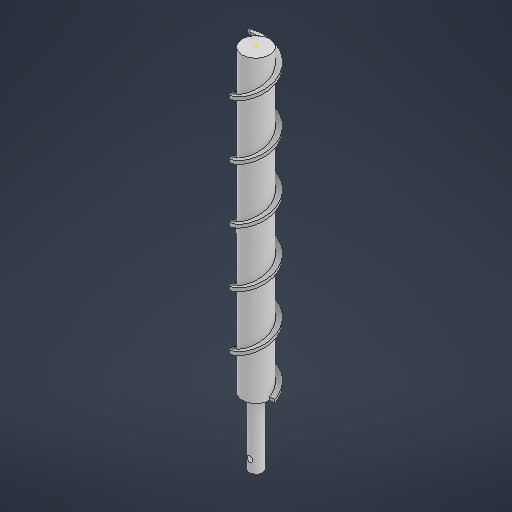
# Autodesk Inventor part: alimentaciion tornillo
Saved by Autodesk Inventor 2026.1 (Build 301233020, 233B)
## iProperties
Created: 2025-12-02
Part Number: alimentaciion tornillo
Material: Genérico
Document SubType Name: Modeling
Designer: benja
Density: 1 g/cm^3
Appearance: Valor por defecto
Author: benja
Autodesk Inventor part; units mm, degrees
ref_plane "YZ Plane" through (0, 0, 0) normal (1, 0, 0) x (0, 1, 0)
ref_plane "XZ Plane" through (0, 0, 0) normal (0, 1, 0) x (-1, 0, 0)
ref_plane "XY Plane" through (0, 0, 0) normal (0, 0, 1) x (1, 0, 0)
sketch "Boceto1" plane through (0, 0, 0) normal (0, 1, 0) x (-1, 0, 0)
  circle A0 centre (0, 0) radius 12.5
  dimension "d0" = 25
  constraints: 1 centre point, 1 coincident
  measures "d0" diameter of A0
extrude "Extrusión1" add sketch "Boceto1" along normal blind 271.2
sketch "Boceto2" plane through (0, 271.2, 0) normal (0, 1, 0) x (1, 0, 0)
  point P0 (0, 0)
sketch "Boceto5" plane through (0, 0, 0) normal (0, 0, 1) x (1, 0, 0)
  line L0 (12.5, 0) -> (-12.5, 0) projected
  line L1 (12.5, 0) -> (21.4, 0)
  line L2 (12.5, 0) -> (21.4, 0)
  line L3 (12.5, 0) -> (21.4, 0) construction
  line L4 (21.4, 0) -> (21.4, 3)
  line L5 (21.4, 3) -> (12.5, 3)
  line L6 (12.5, 3) -> (12.5, 0)
  point P0 (0, 0)
  dimension "d18" = 8.9
  dimension "d19" = 0
  dimension "d20" = 3
  dimension "d21" = 90
  constraints: 12 end point, 3 collinear, 3 perpendicular, 1 horizontal
  measures "d18" distance of L0.start L1.end
  measures "d19" distance between parallel lines of L2 L3
  measures "d20" distance of L1.end L4.end
  measures "d21" angle of L4 L2
sketch3d "Boceto 3D1"
  helix H0 starts at (9.45, 0, 0) axis through (0, 0, 0) along (0, 1, 0) pitch 50 turns 5.424 hand right
sweep "Barrido1" add profiles "Boceto5" path "Boceto 3D1"
sketch "Boceto8" plane through (0, 0, 0) normal (0, -1, 0) x (1, 0, 0)
  arc A0 (-8.2073, -9.4281) -> (-11.1017, -5.7447) centre (0, 0) ccw projected
  circle A1 centre (0, 0) radius 16.95
  circle A2 centre (0, 0) radius 26.0727
  dimension "d35" = 33.9
  constraints: 2 centre point, 2 coincident
  measures "d35" diameter of A1
extrude "Extrusión4" cut sketch "Boceto8" against normal blind 1000.6
sketch "Boceto11" plane through (0, 0, 0) normal (0, 0, 1) x (1, 0, 0)
  circle A0 centre (0, -19.0367) radius 3
  point P0 (0, 0)
  dimension "d44" = 6
  constraints: 1 centre point
  measures "d44" diameter of A0
extrude "Extrusión7" cut sketch "Boceto11" along normal mid plane 30
sketch "Boceto12" plane through (0, 0, 0) normal (0, -1, 0) x (1, 0, 0)
  circle A0 centre (0, 0) radius 6
  dimension "d48" = 12
  constraints: 1 centre point, 1 coincident
  measures "d48" diameter of A0
extrude "Extrusión8" add sketch "Boceto12" along normal blind 60
sketch "Boceto13" plane through (0, 0, 0) normal (0, 0, 1) x (1, 0, 0)
  circle A0 centre (0, -49.1048) radius 2.5
  point P0 (0, 0)
  dimension "d51" = 5
  constraints: 1 centre point
  measures "d51" diameter of A0
extrude "Extrusión9" cut sketch "Boceto13" along normal mid plane 60
